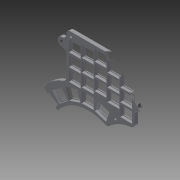
# Autodesk Inventor part: 20kb rebuild Printable Left
Saved by Autodesk Inventor 2015 SP2 (Build 190223200, 223)
## iProperties
Created: 2016-01-05
Part Number: 20kb rebuild Printable Left
Material: Generic
Document SubType Name: Modeling
Designer: Josh
Density: 1 g/cm^3
Appearance: Default
Author: Josh
Autodesk Inventor part; units mm, degrees
(part 1 of 2)
ref_plane "YZ Plane" through (0, 0, 0) normal (1, 0, 0) x (0, 1, 0)
ref_plane "XZ Plane" through (0, 0, 0) normal (0, 1, 0) x (-1, 0, 0)
ref_plane "XY Plane" through (0, 0, 0) normal (0, 0, 1) x (1, 0, 0)
sketch "Sketch1" plane through (0, 0, 0) normal (0, 0, 1) x (1, 0, 0)
  line L0 (4.268, -29.8985) -> (3.518, -29.8985) projected
  line L1 (3.518, -29.8985) -> (3.518, -30.4985) projected
  line L2 (3.518, -30.4985) -> (-10.482, -30.4985) projected
  line L3 (-10.482, -30.4985) -> (-10.482, -29.8985) projected
  line L4 (-10.482, -29.8985) -> (-11.232, -29.8985) projected
  line L5 (-11.232, -29.8985) -> (-11.232, -17.0985) projected
  line L6 (-11.232, -17.0985) -> (-10.482, -17.0985) projected
  line L7 (-10.482, -17.0985) -> (-10.482, -16.4985) projected
  line L8 (-10.482, -16.4985) -> (3.518, -16.4985) projected
  line L9 (3.518, -16.4985) -> (3.518, -17.0985) projected
  line L10 (3.518, -17.0985) -> (4.268, -17.0985) projected
  line L11 (4.268, -17.0985) -> (4.268, -29.8985) projected
  line L12 (26.884, -23.4145) -> (27.5924, -23.661) projected
  line L13 (27.5924, -23.661) -> (23.3854, -35.7499) projected
  line L14 (23.3854, -35.7499) -> (22.6771, -35.5034) projected
  line L15 (22.6771, -35.5034) -> (22.4799, -36.0701) projected
  line L16 (22.4799, -36.0701) -> (9.2576, -31.4687) projected
  line L17 (9.2576, -31.4687) -> (9.4548, -30.902) projected
  line L18 (9.4548, -30.902) -> (8.7465, -30.6555) projected
  line L19 (8.7465, -30.6555) -> (12.9535, -18.5666) projected
  line L20 (12.9535, -18.5666) -> (13.6618, -18.8131) projected
  line L21 (13.6618, -18.8131) -> (13.859, -18.2465) projected
  line L22 (13.859, -18.2465) -> (27.0812, -22.8479) projected
  line L23 (27.0812, -22.8479) -> (26.884, -23.4145) projected
  line L24 (-15.7105, -30.6555) -> (-16.4188, -30.902) projected
  line L25 (-16.4188, -30.902) -> (-16.2216, -31.4687) projected
  line L26 (-16.2216, -31.4687) -> (-29.4438, -36.0701) projected
  line L27 (-29.4438, -36.0701) -> (-29.641, -35.5034) projected
  line L28 (-29.641, -35.5034) -> (-30.3494, -35.7499) projected
  line L29 (-30.3494, -35.7499) -> (-34.5564, -23.661) projected
  line L30 (-34.5564, -23.661) -> (-33.848, -23.4145) projected
  line L31 (-33.848, -23.4145) -> (-34.0452, -22.8479) projected
  line L32 (-34.0452, -22.8479) -> (-20.823, -18.2465) projected
  line L33 (-20.823, -18.2465) -> (-20.6258, -18.8131) projected
  line L34 (-20.6258, -18.8131) -> (-19.9175, -18.5666) projected
  line L35 (-19.9175, -18.5666) -> (-15.7105, -30.6555) projected
  line L36 (-34.3302, -37.9368) -> (-34.9182, -38.4024) projected
  line L37 (-34.9182, -38.4024) -> (-34.5457, -38.8728) projected
  line L38 (-34.5457, -38.8728) -> (-45.521, -47.5643) projected
  line L39 (-45.521, -47.5643) -> (-45.8935, -47.0939) projected
  line L40 (-45.8935, -47.0939) -> (-46.4815, -47.5596) projected
  line L41 (-46.4815, -47.5596) -> (-54.428, -37.525) projected
  line L42 (-54.428, -37.525) -> (-53.84, -37.0594) projected
  line L43 (-53.84, -37.0594) -> (-54.2125, -36.589) projected
  line L44 (-54.2125, -36.589) -> (-43.2372, -27.8975) projected
  line L45 (-43.2372, -27.8975) -> (-42.8647, -28.3679) projected
  line L46 (-42.8647, -28.3679) -> (-42.2768, -27.9022) projected
  line L47 (-42.2768, -27.9022) -> (-34.3302, -37.9368) projected
  line L48 (-49.5224, -50.9334) -> (-49.9247, -51.5664) projected
  line L49 (-49.9247, -51.5664) -> (-49.4183, -51.8882) projected
  line L50 (-49.4183, -51.8882) -> (-56.9272, -63.7041) projected
  line L51 (-56.9272, -63.7041) -> (-57.4336, -63.3823) projected
  line L52 (-57.4336, -63.3823) -> (-57.8359, -64.0153) projected
  line L53 (-57.8359, -64.0153) -> (-68.639, -57.15) projected
  line L54 (-68.639, -57.15) -> (-68.2367, -56.517) projected
  line L55 (-68.2367, -56.517) -> (-68.7431, -56.1952) projected
  line L56 (-68.7431, -56.1952) -> (-61.2342, -44.3793) projected
  line L57 (-61.2342, -44.3793) -> (-60.7278, -44.7011) projected
  line L58 (-60.7278, -44.7011) -> (-60.3256, -44.0681) projected
  line L59 (-60.3256, -44.0681) -> (-49.5224, -50.9334) projected
  line L60 (-15.532, 38.9932) -> (-14.782, 38.9932) projected
  line L61 (-14.782, 38.9932) -> (-14.782, 26.1932) projected
  line L62 (-14.782, 26.1932) -> (-15.532, 26.1932) projected
  line L63 (-15.532, 26.1932) -> (-15.532, 25.5932) projected
  line L64 (-15.532, 25.5932) -> (-29.532, 25.5932) projected
  line L65 (-29.532, 25.5932) -> (-29.532, 26.1932) projected
  line L66 (-29.532, 26.1932) -> (-30.282, 26.1932) projected
  line L67 (-30.282, 26.1932) -> (-30.282, 38.9932) projected
  line L68 (-30.282, 38.9932) -> (-29.532, 38.9932) projected
  line L69 (-29.532, 38.9932) -> (-29.532, 39.5932) projected
  line L70 (-29.532, 39.5932) -> (-15.532, 39.5932) projected
  line L71 (-15.532, 39.5932) -> (-15.532, 38.9932) projected
  line L72 (3.518, 41.3744) -> (4.268, 41.3744) projected
  line L73 (4.268, 41.3744) -> (4.268, 28.5744) projected
  line L74 (4.268, 28.5744) -> (3.518, 28.5744) projected
  line L75 (3.518, 28.5744) -> (3.518, 27.9744) projected
  line L76 (3.518, 27.9744) -> (-10.482, 27.9744) projected
  line L77 (-10.482, 27.9744) -> (-10.482, 28.5744) projected
  line L78 (-10.482, 28.5744) -> (-11.232, 28.5744) projected
  line L79 (-11.232, 28.5744) -> (-11.232, 41.3744) projected
  line L80 (-11.232, 41.3744) -> (-10.482, 41.3744) projected
  line L81 (-10.482, 41.3744) -> (-10.482, 41.9744) projected
  line L82 (-10.482, 41.9744) -> (3.518, 41.9744) projected
  line L83 (3.518, 41.9744) -> (3.518, 41.3744) projected
  line L84 (60.668, 31.8494) -> (61.418, 31.8494) projected
  line L85 (61.418, 31.8494) -> (61.418, 19.0494) projected
  line L86 (61.418, 19.0494) -> (60.668, 19.0494) projected
  line L87 (60.668, 19.0494) -> (60.668, 18.4494) projected
  line L88 (60.668, 18.4494) -> (46.668, 18.4494) projected
  line L89 (46.668, 18.4494) -> (46.668, 19.0494) projected
  line L90 (46.668, 19.0494) -> (45.918, 19.0494) projected
  line L91 (45.918, 19.0494) -> (45.918, 31.8494) projected
  line L92 (45.918, 31.8494) -> (46.668, 31.8494) projected
  line L93 (46.668, 31.8494) -> (46.668, 32.4494) projected
  line L94 (46.668, 32.4494) -> (60.668, 32.4494) projected
  line L95 (60.668, 32.4494) -> (60.668, 31.8494) projected
  line L96 (22.568, 46.1369) -> (23.318, 46.1369) projected
  line L97 (23.318, 46.1369) -> (23.318, 33.3369) projected
  line L98 (23.318, 33.3369) -> (22.568, 33.3369) projected
  line L99 (22.568, 33.3369) -> (22.568, 32.7369) projected
  line L100 (22.568, 32.7369) -> (8.568, 32.7369) projected
  line L101 (8.568, 32.7369) -> (8.568, 33.3369) projected
  line L102 (8.568, 33.3369) -> (7.818, 33.3369) projected
  line L103 (7.818, 33.3369) -> (7.818, 46.1369) projected
  line L104 (7.818, 46.1369) -> (8.568, 46.1369) projected
  line L105 (8.568, 46.1369) -> (8.568, 46.7369) projected
  line L106 (8.568, 46.7369) -> (22.568, 46.7369) projected
  line L107 (22.568, 46.7369) -> (22.568, 46.1369) projected
  line L108 (41.618, 41.3744) -> (42.368, 41.3744) projected
  line L109 (42.368, 41.3744) -> (42.368, 28.5744) projected
  line L110 (42.368, 28.5744) -> (41.618, 28.5744) projected
  line L111 (41.618, 28.5744) -> (41.618, 27.9744) projected
  line L112 (41.618, 27.9744) -> (27.618, 27.9744) projected
  line L113 (27.618, 27.9744) -> (27.618, 28.5744) projected
  line L114 (27.618, 28.5744) -> (26.868, 28.5744) projected
  line L115 (26.868, 28.5744) -> (26.868, 41.3744) projected
  line L116 (26.868, 41.3744) -> (27.618, 41.3744) projected
  line L117 (27.618, 41.3744) -> (27.618, 41.9744) projected
  line L118 (27.618, 41.9744) -> (41.618, 41.9744) projected
  line L119 (41.618, 41.9744) -> (41.618, 41.3744) projected
  line L120 (-15.532, 19.9432) -> (-14.782, 19.9432) projected
  line L121 (-14.782, 19.9432) -> (-14.782, 7.1432) projected
  line L122 (-14.782, 7.1432) -> (-15.532, 7.1432) projected
  line L123 (-15.532, 7.1432) -> (-15.532, 6.5432) projected
  line L124 (-15.532, 6.5432) -> (-29.532, 6.5432) projected
  line L125 (-29.532, 6.5432) -> (-29.532, 7.1432) projected
  line L126 (-29.532, 7.1432) -> (-30.282, 7.1432) projected
  line L127 (-30.282, 7.1432) -> (-30.282, 19.9432) projected
  line L128 (-30.282, 19.9432) -> (-29.532, 19.9432) projected
  line L129 (-29.532, 19.9432) -> (-29.532, 20.5432) projected
  line L130 (-29.532, 20.5432) -> (-15.532, 20.5432) projected
  line L131 (-15.532, 20.5432) -> (-15.532, 19.9432) projected
  line L132 (3.518, 22.3244) -> (4.268, 22.3244) projected
  line L133 (4.268, 22.3244) -> (4.268, 9.5244) projected
  line L134 (4.268, 9.5244) -> (3.518, 9.5244) projected
  line L135 (3.518, 9.5244) -> (3.518, 8.9244) projected
  line L136 (3.518, 8.9244) -> (-10.482, 8.9244) projected
  line L137 (-10.482, 8.9244) -> (-10.482, 9.5244) projected
  line L138 (-10.482, 9.5244) -> (-11.232, 9.5244) projected
  line L139 (-11.232, 9.5244) -> (-11.232, 22.3244) projected
  line L140 (-11.232, 22.3244) -> (-10.482, 22.3244) projected
  line L141 (-10.482, 22.3244) -> (-10.482, 22.9244) projected
  line L142 (-10.482, 22.9244) -> (3.518, 22.9244) projected
  line L143 (3.518, 22.9244) -> (3.518, 22.3244) projected
  line L144 (60.668, 12.7994) -> (61.418, 12.7994) projected
  line L145 (61.418, 12.7994) -> (61.418, -0.0006) projected
  line L146 (61.418, -0.0006) -> (60.668, -0.0006) projected
  line L147 (60.668, -0.0006) -> (60.668, -0.6006) projected
  line L148 (60.668, -0.6006) -> (46.668, -0.6006) projected
  line L149 (46.668, -0.6006) -> (46.668, -0.0006) projected
  line L150 (46.668, -0.0006) -> (45.918, -0.0006) projected
  line L151 (45.918, -0.0006) -> (45.918, 12.7994) projected
  line L152 (45.918, 12.7994) -> (46.668, 12.7994) projected
  line L153 (46.668, 12.7994) -> (46.668, 13.3994) projected
  line L154 (46.668, 13.3994) -> (60.668, 13.3994) projected
  line L155 (60.668, 13.3994) -> (60.668, 12.7994) projected
  line L156 (22.568, 27.0869) -> (23.318, 27.0869) projected
  line L157 (23.318, 27.0869) -> (23.318, 14.2869) projected
  line L158 (23.318, 14.2869) -> (22.568, 14.2869) projected
  line L159 (22.568, 14.2869) -> (22.568, 13.6869) projected
  line L160 (22.568, 13.6869) -> (8.568, 13.6869) projected
  line L161 (8.568, 13.6869) -> (8.568, 14.2869) projected
  line L162 (8.568, 14.2869) -> (7.818, 14.2869) projected
  line L163 (7.818, 14.2869) -> (7.818, 27.0869) projected
  line L164 (7.818, 27.0869) -> (8.568, 27.0869) projected
  line L165 (8.568, 27.0869) -> (8.568, 27.6869) projected
  line L166 (8.568, 27.6869) -> (22.568, 27.6869) projected
  line L167 (22.568, 27.6869) -> (22.568, 27.0869) projected
  line L168 (41.618, 22.3244) -> (42.368, 22.3244) projected
  line L169 (42.368, 22.3244) -> (42.368, 9.5244) projected
  line L170 (42.368, 9.5244) -> (41.618, 9.5244) projected
  line L171 (41.618, 9.5244) -> (41.618, 8.9244) projected
  line L172 (41.618, 8.9244) -> (27.618, 8.9244) projected
  line L173 (27.618, 8.9244) -> (27.618, 9.5244) projected
  line L174 (27.618, 9.5244) -> (26.868, 9.5244) projected
  line L175 (26.868, 9.5244) -> (26.868, 22.3244) projected
  line L176 (26.868, 22.3244) -> (27.618, 22.3244) projected
  line L177 (27.618, 22.3244) -> (27.618, 22.9244) projected
  line L178 (27.618, 22.9244) -> (41.618, 22.9244) projected
  line L179 (41.618, 22.9244) -> (41.618, 22.3244) projected
  line L180 (42.368, -9.5256) -> (41.618, -9.5256) projected
  line L181 (41.618, -9.5256) -> (41.618, -10.1256) projected
  line L182 (41.618, -10.1256) -> (27.618, -10.1256) projected
  line L183 (27.618, -10.1256) -> (27.618, -9.5256) projected
  line L184 (27.618, -9.5256) -> (26.868, -9.5256) projected
  line L185 (26.868, -9.5256) -> (26.868, 3.2744) projected
  line L186 (26.868, 3.2744) -> (27.618, 3.2744) projected
  line L187 (27.618, 3.2744) -> (27.618, 3.8744) projected
  line L188 (27.618, 3.8744) -> (41.618, 3.8744) projected
  line L189 (41.618, 3.8744) -> (41.618, 3.2744) projected
  line L190 (41.618, 3.2744) -> (42.368, 3.2744) projected
  line L191 (42.368, 3.2744) -> (42.368, -9.5256) projected
  line L192 (23.318, -4.7631) -> (22.568, -4.7631) projected
  line L193 (22.568, -4.7631) -> (22.568, -5.3631) projected
  line L194 (22.568, -5.3631) -> (8.568, -5.3631) projected
  line L195 (8.568, -5.3631) -> (8.568, -4.7631) projected
  line L196 (8.568, -4.7631) -> (7.818, -4.7631) projected
  line L197 (7.818, -4.7631) -> (7.818, 8.0369) projected
  line L198 (7.818, 8.0369) -> (8.568, 8.0369) projected
  line L199 (8.568, 8.0369) -> (8.568, 8.6369) projected
  line L200 (8.568, 8.6369) -> (22.568, 8.6369) projected
  line L201 (22.568, 8.6369) -> (22.568, 8.0369) projected
  line L202 (22.568, 8.0369) -> (23.318, 8.0369) projected
  line L203 (23.318, 8.0369) -> (23.318, -4.7631) projected
  line L204 (61.418, -19.0506) -> (60.668, -19.0506) projected
  line L205 (60.668, -19.0506) -> (60.668, -19.6506) projected
  line L206 (60.668, -19.6506) -> (46.668, -19.6506) projected
  line L207 (46.668, -19.6506) -> (46.668, -19.0506) projected
  line L208 (46.668, -19.0506) -> (45.918, -19.0506) projected
  line L209 (45.918, -19.0506) -> (45.918, -6.2506) projected
  line L210 (45.918, -6.2506) -> (46.668, -6.2506) projected
  line L211 (46.668, -6.2506) -> (46.668, -5.6506) projected
  line L212 (46.668, -5.6506) -> (60.668, -5.6506) projected
  line L213 (60.668, -5.6506) -> (60.668, -6.2506) projected
  line L214 (60.668, -6.2506) -> (61.418, -6.2506) projected
  line L215 (61.418, -6.2506) -> (61.418, -19.0506) projected
  line L216 (4.268, -9.5256) -> (3.518, -9.5256) projected
  line L217 (3.518, -9.5256) -> (3.518, -10.1256) projected
  line L218 (3.518, -10.1256) -> (-10.482, -10.1256) projected
  line L219 (-10.482, -10.1256) -> (-10.482, -9.5256) projected
  line L220 (-10.482, -9.5256) -> (-11.232, -9.5256) projected
  line L221 (-11.232, -9.5256) -> (-11.232, 3.2744) projected
  line L222 (-11.232, 3.2744) -> (-10.482, 3.2744) projected
  line L223 (-10.482, 3.2744) -> (-10.482, 3.8744) projected
  line L224 (-10.482, 3.8744) -> (3.518, 3.8744) projected
  line L225 (3.518, 3.8744) -> (3.518, 3.2744) projected
  line L226 (3.518, 3.2744) -> (4.268, 3.2744) projected
  line L227 (4.268, 3.2744) -> (4.268, -9.5256) projected
  line L228 (-14.782, -11.9068) -> (-15.532, -11.9068) projected
  line L229 (-15.532, -11.9068) -> (-15.532, -12.5068) projected
  line L230 (-15.532, -12.5068) -> (-29.532, -12.5068) projected
  line L231 (-29.532, -12.5068) -> (-29.532, -11.9068) projected
  line L232 (-29.532, -11.9068) -> (-30.282, -11.9068) projected
  line L233 (-30.282, -11.9068) -> (-30.282, 0.8932) projected
  line L234 (-30.282, 0.8932) -> (-29.532, 0.8932) projected
  line L235 (-29.532, 0.8932) -> (-29.532, 1.4932) projected
  line L236 (-29.532, 1.4932) -> (-15.532, 1.4932) projected
  line L237 (-15.532, 1.4932) -> (-15.532, 0.8932) projected
  line L238 (-15.532, 0.8932) -> (-14.782, 0.8932) projected
  line L239 (-14.782, 0.8932) -> (-14.782, -11.9068) projected
  arc A0 (66.368, 46.0869) -> (60.018, 52.4369) centre (60.018, 46.0869) ccw projected
  line L240 (-28.882, 52.4369) -> (60.018, 52.4369) projected
  arc A1 (-28.882, 52.4369) -> (-35.232, 46.0869) centre (-28.882, 46.0869) ccw projected
  line L241 (-35.232, -10.3249) -> (-35.232, 46.0869) projected
  arc A2 (-39.5057, -16.3259) -> (-35.232, -10.3249) centre (-41.582, -10.3249) ccw projected
  arc A3 (-39.5057, -16.3259) -> (-76.6111, -57.9488) centre (-20.8194, -70.3346) ccw projected
  arc A4 (22.0394, -41.2849) -> (29.0899, -40.1547) centre (24.7335, -35.5347) ccw projected
  arc A5 (60.6824, -25.6489) -> (29.0899, -40.1547) centre (66.368, -79.6875) ccw projected
  arc A6 (60.6824, -25.6489) -> (66.368, -19.3337) centre (60.018, -19.3337) ccw projected
  line L242 (66.368, 46.0869) -> (66.368, -19.3337) projected
  line L243 (-15.5241, 49.2404) -> (-15.124, 49.2404) construction
  line L244 (-15.124, 49.2404) -> (-16.3541, 46.1109) construction
  line L245 (-16.3541, 46.1109) -> (-16.7666, 46.1109) construction
  line L246 (-16.7666, 46.1109) -> (-16.3565, 47.0643) construction
  line L247 (-16.3565, 47.0643) -> (-17.1865, 49.2404) construction
  line L248 (-17.1865, 49.2404) -> (-16.7715, 49.2404) construction
  line L249 (-16.7715, 49.2404) -> (-16.1466, 47.546) construction
  line L250 (-16.1466, 47.546) -> (-15.5241, 49.2404) construction
  spline S0 degree 2 poles (-20.9606, 46.9729) (-21.0693, 46.9433) (-21.2916, 46.9087) (-21.388, 46.9087) knots 0 0 0 1 2 2 2 construction
  spline S1 degree 2 poles (-21.388, 46.9087) (-21.7016, 46.9087) (-22.0549, 47.2669) (-22.0549, 47.6546) knots 0 0 0 1 2 2 2 construction
  line L251 (-22.0549, 47.6546) -> (-22.0549, 48.9218) construction
  line L252 (-22.0549, 48.9218) -> (-22.3142, 48.9218) construction
  line L253 (-22.3142, 48.9218) -> (-22.3142, 49.2404) construction
  line L254 (-22.3142, 49.2404) -> (-22.0549, 49.2404) construction
  line L255 (-22.0549, 49.2404) -> (-22.0549, 49.8974) construction
  line L256 (-22.0549, 49.8974) -> (-21.6695, 49.8974) construction
  line L257 (-21.6695, 49.8974) -> (-21.6695, 49.2404) construction
  line L258 (-21.6695, 49.2404) -> (-20.9606, 49.2404) construction
  line L259 (-20.9606, 49.2404) -> (-20.9606, 48.9218) construction
  line L260 (-20.9606, 48.9218) -> (-21.6695, 48.9218) construction
  line L261 (-21.6695, 48.9218) -> (-21.6695, 47.8325) construction
  spline S2 degree 2 poles (-21.6695, 47.8325) (-21.6695, 47.6596) (-21.6572, 47.4694) (-21.6152, 47.3879) knots 0 0 0 1 2 2 2 construction
  spline S3 degree 2 poles (-21.6152, 47.3879) (-21.5806, 47.3163) (-21.425, 47.2446) (-21.2916, 47.2446) knots 0 0 0 1 2 2 2 construction
  spline S4 degree 2 poles (-21.2916, 47.2446) (-21.1978, 47.2446) (-21.0224, 47.3014) (-20.9829, 47.3187) knots 0 0 0 1 2 2 2 construction
  line L262 (-20.9829, 47.3187) -> (-20.9606, 47.3187) construction
  line L263 (-20.9606, 47.3187) -> (-20.9606, 46.9729) construction
  line L264 (-27.4568, 46.9532) -> (-27.8619, 46.9532) construction
  line L265 (-27.8619, 46.9532) -> (-27.8619, 49.6405) construction
  line L266 (-27.8619, 49.6405) -> (-28.8845, 49.6405) construction
  line L267 (-28.8845, 49.6405) -> (-28.8845, 50.0012) construction
  line L268 (-28.8845, 50.0012) -> (-26.4342, 50.0012) construction
  line L269 (-26.4342, 50.0012) -> (-26.4342, 49.6405) construction
  line L270 (-26.4342, 49.6405) -> (-27.4568, 49.6405) construction
  line L271 (-27.4568, 49.6405) -> (-27.4568, 46.9532) construction
  spline S5 degree 2 poles (53.9938, 46.8371) (53.8851, 46.8074) (53.6628, 46.7728) (53.5664, 46.7728) knots 0 0 0 1 2 2 2 construction
  spline S6 degree 2 poles (53.5664, 46.7728) (53.2527, 46.7728) (52.8995, 47.131) (52.8995, 47.5188) knots 0 0 0 1 2 2 2 construction
  line L272 (52.8995, 47.5188) -> (52.8995, 48.7859) construction
  line L273 (52.8995, 48.7859) -> (52.6402, 48.7859) construction
  line L274 (52.6402, 48.7859) -> (52.6402, 49.1045) construction
  line L275 (52.6402, 49.1045) -> (52.8995, 49.1045) construction
  line L276 (52.8995, 49.1045) -> (52.8995, 49.7616) construction
  line L277 (52.8995, 49.7616) -> (53.2849, 49.7616) construction
  line L278 (53.2849, 49.7616) -> (53.2849, 49.1045) construction
  line L279 (53.2849, 49.1045) -> (53.9938, 49.1045) construction
  line L280 (53.9938, 49.1045) -> (53.9938, 48.7859) construction
  line L281 (53.9938, 48.7859) -> (53.2849, 48.7859) construction
  line L282 (53.2849, 48.7859) -> (53.2849, 47.6966) construction
  spline S7 degree 2 poles (53.2849, 47.6966) (53.2849, 47.5237) (53.2972, 47.3335) (53.3392, 47.252) knots 0 0 0 1 2 2 2 construction
  spline S8 degree 2 poles (53.3392, 47.252) (53.3738, 47.1804) (53.5294, 47.1088) (53.6628, 47.1088) knots 0 0 0 1 2 2 2 construction
  spline S9 degree 2 poles (53.6628, 47.1088) (53.7566, 47.1088) (53.932, 47.1656) (53.9715, 47.1829) knots 0 0 0 1 2 2 2 construction
  line L283 (53.9715, 47.1829) -> (53.9938, 47.1829) construction
  line L284 (53.9938, 47.1829) -> (53.9938, 46.8371) construction
  line L285 (52.3092, 49.1045) -> (52.3092, 46.8173) construction
  line L286 (52.3092, 46.8173) -> (51.9239, 46.8173) construction
  line L287 (51.9239, 46.8173) -> (51.9239, 49.1045) construction
  line L288 (51.9239, 49.1045) -> (52.3092, 49.1045) construction
  spline S10 degree 2 poles (48.7376, 47.0347) (48.5918, 46.8914) (48.2065, 46.7531) (47.9249, 46.7531) knots 0 0 0 1 2 2 2 construction
  spline S11 degree 2 poles (47.9249, 46.7531) (47.6557, 46.7531) (47.2555, 46.8939) (47.1148, 47.0347) knots 0 0 0 1 2 2 2 construction
  spline S12 degree 2 poles (47.1148, 47.0347) (46.9542, 47.1927) (46.8233, 47.6374) (46.8233, 47.9634) knots 0 0 0 1 2 2 2 construction
  line L289 (46.8233, 47.9634) -> (46.8233, 49.8653) construction
  line L290 (46.8233, 49.8653) -> (47.2284, 49.8653) construction
  line L291 (47.2284, 49.8653) -> (47.2284, 47.9634) construction
  spline S13 degree 2 poles (47.2284, 47.9634) (47.2284, 47.751) (47.2827, 47.4645) (47.3593, 47.3484) knots 0 0 0 1 2 2 2 construction
  spline S14 degree 2 poles (47.3593, 47.3484) (47.4408, 47.2249) (47.7224, 47.0989) (47.9249, 47.0989) knots 0 0 0 1 2 2 2 construction
  spline S15 degree 2 poles (47.9249, 47.0989) (48.1151, 47.0989) (48.4115, 47.2249) (48.493, 47.3484) knots 0 0 0 1 2 2 2 construction
  spline S16 degree 2 poles (48.493, 47.3484) (48.5696, 47.4645) (48.6239, 47.7485) (48.6239, 47.9535) knots 0 0 0 1 2 2 2 construction
  line L292 (48.6239, 47.9535) -> (48.6239, 49.8653) construction
  line L293 (48.6239, 49.8653) -> (49.029, 49.8653) construction
  line L294 (49.029, 49.8653) -> (49.029, 47.9634) construction
  spline S17 degree 2 poles (49.029, 47.9634) (49.029, 47.6448) (48.9006, 47.1903) (48.7376, 47.0347) knots 0 0 0 1 2 2 2 construction
  line L295 (44.9634, 50.0012) -> (44.9634, 46.8173) construction
  line L296 (44.9634, 46.8173) -> (44.5781, 46.8173) construction
  line L297 (44.5781, 46.8173) -> (44.5781, 47.0495) construction
  spline S18 degree 2 poles (44.5781, 47.0495) (44.4891, 46.9754) (44.3582, 46.8766) (44.2693, 46.8346) knots 0 0 0 1 2 2 2 construction
  spline S19 degree 2 poles (44.2693, 46.8346) (44.1878, 46.7951) (44.0124, 46.7531) (43.8963, 46.7531) knots 0 0 0 1 2 2 2 construction
  spline S20 degree 2 poles (43.8963, 46.7531) (43.7086, 46.7531) (43.3924, 46.9087) (43.2813, 47.0594) knots 0 0 0 1 2 2 2 construction
  spline S21 degree 2 poles (43.2813, 47.0594) (43.1701, 47.21) (43.0466, 47.6546) (43.0466, 47.9436) knots 0 0 0 1 2 2 2 construction
  spline S22 degree 2 poles (43.0466, 47.9436) (43.0466, 48.245) (43.2023, 48.6846) (43.3381, 48.8501) knots 0 0 0 1 2 2 2 construction
  spline S23 degree 2 poles (43.3381, 48.8501) (43.4641, 48.9983) (43.8173, 49.1688) (44.0124, 49.1688) knots 0 0 0 1 2 2 2 construction
  spline S24 degree 2 poles (44.0124, 49.1688) (44.1828, 49.1688) (44.4373, 49.0922) (44.5781, 49.0132) knots 0 0 0 1 2 2 2 construction
  line L298 (44.5781, 49.0132) -> (44.5781, 50.0012) construction
  line L299 (44.5781, 50.0012) -> (44.9634, 50.0012) construction
  line L300 (34.2089, 49.1045) -> (34.6091, 49.1045) construction
  line L301 (34.6091, 49.1045) -> (33.379, 45.975) construction
  line L302 (33.379, 45.975) -> (32.9665, 45.975) construction
  line L303 (32.9665, 45.975) -> (33.3765, 46.9285) construction
  line L304 (33.3765, 46.9285) -> (32.5466, 49.1045) construction
  line L305 (32.5466, 49.1045) -> (32.9616, 49.1045) construction
  line L306 (32.9616, 49.1045) -> (33.5865, 47.4101) construction
  line L307 (33.5865, 47.4101) -> (34.2089, 49.1045) construction
  spline S25 degree 2 poles (32.0328, 46.8297) (31.9217, 46.7975) (31.7389, 46.7654) (31.6006, 46.7654) knots 0 0 0 1 2 2 2 construction
  spline S26 degree 2 poles (31.6006, 46.7654) (31.0522, 46.7654) (30.4496, 47.3805) (30.4496, 47.9486) knots 0 0 0 1 2 2 2 construction
  spline S27 degree 2 poles (30.4496, 47.9486) (30.4496, 48.5068) (31.035, 49.1688) (31.5067, 49.1688) knots 0 0 0 1 2 2 2 construction
  spline S28 degree 2 poles (31.5067, 49.1688) (31.7191, 49.1688) (32.0477, 49.0453) (32.1687, 48.9144) knots 0 0 0 1 2 2 2 construction
  spline S29 degree 2 poles (32.1687, 48.9144) (32.2922, 48.7834) (32.4231, 48.4055) (32.4231, 48.1314) knots 0 0 0 1 2 2 2 construction
  line L308 (32.4231, 48.1314) -> (32.4231, 47.9214) construction
  line L309 (32.4231, 47.9214) -> (30.8398, 47.9214) construction
  spline S30 degree 2 poles (30.8398, 47.9214) (30.8398, 47.5237) (31.24, 47.1014) (31.5956, 47.1014) knots 0 0 0 1 2 2 2 construction
  spline S31 degree 2 poles (31.5956, 47.1014) (31.7216, 47.1014) (31.9661, 47.1582) (32.0649, 47.2026) knots 0 0 0 1 2 2 2 construction
  spline S32 degree 2 poles (32.0649, 47.2026) (32.1687, 47.252) (32.312, 47.3385) (32.3589, 47.378) knots 0 0 0 1 2 2 2 construction
  line L310 (32.3589, 47.378) -> (32.3811, 47.378) construction
  line L311 (32.3811, 47.378) -> (32.3811, 46.9581) construction
  spline S33 degree 2 poles (32.3811, 46.9581) (32.3144, 46.9309) (32.1119, 46.8519) (32.0328, 46.8297) knots 0 0 0 1 2 2 2 construction
  line L312 (29.0589, 48.5043) -> (30.3952, 46.8173) construction
  line L313 (30.3952, 46.8173) -> (29.8691, 46.8173) construction
  line L314 (29.8691, 46.8173) -> (28.7551, 48.2351) construction
  line L315 (28.7551, 48.2351) -> (28.5773, 48.035) construction
  line L316 (28.5773, 48.035) -> (28.5773, 46.8173) construction
  line L317 (28.5773, 46.8173) -> (28.1722, 46.8173) construction
  line L318 (28.1722, 46.8173) -> (28.1722, 49.8653) construction
  line L319 (28.1722, 49.8653) -> (28.5773, 49.8653) construction
  line L320 (28.5773, 49.8653) -> (28.5773, 48.4648) construction
  line L321 (28.5773, 48.4648) -> (29.8271, 49.8653) construction
  line L322 (29.8271, 49.8653) -> (30.3211, 49.8653) construction
  line L323 (30.3211, 49.8653) -> (29.0589, 48.5043) construction
  spline S34 degree 2 poles (35.9849, 49.1688) (36.3727, 49.1688) (36.8173, 48.5488) (36.8173, 47.998) knots 0 0 0 1 2 2 2 construction
  spline S35 degree 2 poles (36.8173, 47.998) (36.8173, 47.4373) (36.2739, 46.7531) (35.8638, 46.7531) knots 0 0 0 1 2 2 2 construction
  spline S36 degree 2 poles (35.8638, 46.7531) (35.6786, 46.7531) (35.4143, 46.8445) (35.2859, 46.9235) knots 0 0 0 1 2 2 2 construction
  line L324 (35.2859, 46.9235) -> (35.2612, 46.8173) construction
  line L325 (35.2612, 46.8173) -> (34.9005, 46.8173) construction
  line L326 (34.9005, 46.8173) -> (34.9005, 50.0012) construction
  line L327 (34.9005, 50.0012) -> (35.2859, 50.0012) construction
  line L328 (35.2859, 50.0012) -> (35.2859, 48.865) construction
  spline S37 degree 2 poles (35.2859, 48.865) (35.4316, 48.9959) (35.77, 49.1688) (35.9849, 49.1688) knots 0 0 0 1 2 2 2 construction
  spline S38 degree 2 poles (38.077, 49.1688) (38.5413, 49.1688) (39.0971, 48.5364) (39.0971, 47.9609) knots 0 0 0 1 2 2 2 construction
  spline S39 degree 2 poles (39.0971, 47.9609) (39.0971, 47.3829) (38.5413, 46.7531) (38.077, 46.7531) knots 0 0 0 1 2 2 2 construction
  spline S40 degree 2 poles (38.077, 46.7531) (37.6003, 46.7531) (37.0544, 47.4027) (37.0544, 47.9609) knots 0 0 0 1 2 2 2 construction
  spline S41 degree 2 poles (37.0544, 47.9609) (37.0544, 48.534) (37.6175, 49.1688) (38.077, 49.1688) knots 0 0 0 1 2 2 2 construction
  line L329 (40.7668, 46.8173) -> (40.7668, 47.0594) construction
  spline S42 degree 2 poles (40.7668, 47.0594) (40.7199, 47.0248) (40.5618, 46.9013) (40.4877, 46.8642) knots 0 0 0 1 2 2 2 construction
  spline S43 degree 2 poles (40.4877, 46.8642) (40.3864, 46.8099) (40.1962, 46.7531) (40.0233, 46.7531) knots 0 0 0 1 2 2 2 construction
  spline S44 degree 2 poles (40.0233, 46.7531) (39.8826, 46.7531) (39.6281, 46.8593) (39.5318, 46.9556) knots 0 0 0 1 2 2 2 construction
  spline S45 degree 2 poles (39.5318, 46.9556) (39.4404, 47.0495) (39.3293, 47.3261) (39.3293, 47.4793) knots 0 0 0 1 2 2 2 construction
  spline S46 degree 2 poles (39.3293, 47.4793) (39.3293, 47.7164) (39.5293, 48.0523) (39.7467, 48.1486) knots 0 0 0 1 2 2 2 construction
  spline S47 degree 2 poles (39.7467, 48.1486) (39.9394, 48.2376) (40.463, 48.3043) (40.7668, 48.3215) knots 0 0 0 1 2 2 2 construction
  line L330 (40.7668, 48.3215) -> (40.7668, 48.3956) construction
  spline S48 degree 2 poles (40.7668, 48.3956) (40.7668, 48.529) (40.6853, 48.6945) (40.6112, 48.7414) knots 0 0 0 1 2 2 2 construction
  spline S49 degree 2 poles (40.6112, 48.7414) (40.5371, 48.7884) (40.3247, 48.818) (40.2111, 48.818) knots 0 0 0 1 2 2 2 construction
  spline S50 degree 2 poles (40.2111, 48.818) (40.0777, 48.818) (39.7171, 48.739) (39.5367, 48.6624) knots 0 0 0 1 2 2 2 construction
  line L331 (39.5367, 48.6624) -> (39.5145, 48.6624) construction
  line L332 (39.5145, 48.6624) -> (39.5145, 49.0551) construction
  spline S51 degree 2 poles (39.5145, 49.0551) (39.6207, 49.0848) (40.0184, 49.1589) (40.2135, 49.1589) knots 0 0 0 1 2 2 2 construction
  spline S52 degree 2 poles (40.2135, 49.1589) (40.4507, 49.1589) (40.7742, 49.0848) (40.9027, 48.9885) knots 0 0 0 1 2 2 2 construction
  spline S53 degree 2 poles (40.9027, 48.9885) (41.0286, 48.8946) (41.1521, 48.5957) (41.1521, 48.3808) knots 0 0 0 1 2 2 2 construction
  line L333 (41.1521, 48.3808) -> (41.1521, 46.8173) construction
  line L334 (41.1521, 46.8173) -> (40.7668, 46.8173) construction
  line L335 (42.9059, 49.0922) -> (42.9059, 48.692) construction
  line L336 (42.9059, 48.692) -> (42.8861, 48.692) construction
  spline S54 degree 2 poles (42.8861, 48.692) (42.8416, 48.7044) (42.7453, 48.7093) (42.6786, 48.7093) knots 0 0 0 1 2 2 2 construction
  spline S55 degree 2 poles (42.6786, 48.7093) (42.523, 48.7093) (42.2167, 48.5735) (42.0784, 48.4401) knots 0 0 0 1 2 2 2 construction
  line L337 (42.0784, 48.4401) -> (42.0784, 46.8173) construction
  line L338 (42.0784, 46.8173) -> (41.6931, 46.8173) construction
  line L339 (41.6931, 46.8173) -> (41.6931, 49.1045) construction
  line L340 (41.6931, 49.1045) -> (42.0784, 49.1045) construction
  line L341 (42.0784, 49.1045) -> (42.0784, 48.7637) construction
  spline S56 degree 2 poles (42.0784, 48.7637) (42.2883, 48.9514) (42.602, 49.1045) (42.7502, 49.1045) knots 0 0 0 1 2 2 2 construction
  spline S57 degree 2 poles (42.7502, 49.1045) (42.8095, 49.1045) (42.8688, 49.0996) (42.9059, 49.0922) knots 0 0 0 1 2 2 2 construction
  line L342 (51.3755, 48.3018) -> (51.3755, 46.8173) construction
  line L343 (51.3755, 46.8173) -> (50.9902, 46.8173) construction
  line L344 (50.9902, 46.8173) -> (50.9902, 48.1215) construction
  spline S58 degree 2 poles (50.9902, 48.1215) (50.9902, 48.2796) (50.9606, 48.5513) (50.9161, 48.6328) knots 0 0 0 1 2 2 2 construction
  spline S59 degree 2 poles (50.9161, 48.6328) (50.8692, 48.7192) (50.7012, 48.8032) (50.558, 48.8032) knots 0 0 0 1 2 2 2 construction
  spline S60 degree 2 poles (50.558, 48.8032) (50.4147, 48.8032) (50.1109, 48.6501) (49.9652, 48.5266) knots 0 0 0 1 2 2 2 construction
  line L345 (49.9652, 48.5266) -> (49.9652, 46.8173) construction
  line L346 (49.9652, 46.8173) -> (49.5798, 46.8173) construction
  line L347 (49.5798, 46.8173) -> (49.5798, 49.1045) construction
  line L348 (49.5798, 49.1045) -> (49.9652, 49.1045) construction
  line L349 (49.9652, 49.1045) -> (49.9652, 48.8501) construction
  spline S61 degree 2 poles (49.9652, 48.8501) (50.1381, 49.0057) (50.4715, 49.1688) (50.6592, 49.1688) knots 0 0 0 1 2 2 2 construction
  spline S62 degree 2 poles (50.6592, 49.1688) (50.9952, 49.1688) (51.3755, 48.7242) (51.3755, 48.3018) knots 0 0 0 1 2 2 2 construction
  line L350 (52.3364, 49.8851) -> (52.3364, 49.4849) construction
  line L351 (52.3364, 49.4849) -> (51.8992, 49.4849) construction
  line L352 (51.8992, 49.4849) -> (51.8992, 49.8851) construction
  line L353 (51.8992, 49.8851) -> (52.3364, 49.8851) construction
  spline S63 degree 2 poles (56.4539, 49.9271) (56.9553, 49.9271) (57.4271, 49.1367) (57.4271, 48.3413) knots 0 0 0 1 2 2 2 construction
  spline S64 degree 2 poles (57.4271, 48.3413) (57.4271, 47.5213) (56.9504, 46.7531) (56.4539, 46.7531) knots 0 0 0 1 2 2 2 construction
  spline S65 degree 2 poles (56.4539, 46.7531) (55.95, 46.7531) (55.4782, 47.5361) (55.4782, 48.3388) knots 0 0 0 1 2 2 2 construction
  spline S66 degree 2 poles (55.4782, 48.3388) (55.4782, 49.1638) (55.9549, 49.9271) (56.4539, 49.9271) knots 0 0 0 1 2 2 2 construction
  line L354 (59.697, 47.1705) -> (59.697, 46.8173) construction
  line L355 (59.697, 46.8173) -> (57.8173, 46.8173) construction
  line L356 (57.8173, 46.8173) -> (57.8173, 47.2496) construction
  spline S67 degree 2 poles (57.8173, 47.2496) (58.0199, 47.4398) (58.3805, 47.793) (58.5534, 47.9832) knots 0 0 0 1 2 2 2 construction
  spline S68 degree 2 poles (58.5534, 47.9832) (58.9017, 48.366) (59.1561, 48.8254) (59.1561, 49.07) knots 0 0 0 1 2 2 2 construction
  spline S69 degree 2 poles (59.1561, 49.07) (59.1561, 49.1984) (59.077, 49.3911) (59.0054, 49.4528) knots 0 0 0 1 2 2 2 construction
  spline S70 degree 2 poles (59.0054, 49.4528) (58.9338, 49.5146) (58.7461, 49.5763) (58.6324, 49.5763) knots 0 0 0 1 2 2 2 construction
  spline S71 degree 2 poles (58.6324, 49.5763) (58.5238, 49.5763) (58.3015, 49.522) (58.2002, 49.48) knots 0 0 0 1 2 2 2 construction
  spline S72 degree 2 poles (58.2002, 49.48) (58.1137, 49.4454) (57.9532, 49.3466) (57.9038, 49.312) knots 0 0 0 1 2 2 2 construction
  line L357 (57.9038, 49.312) -> (57.8816, 49.312) construction
  line L358 (57.8816, 49.312) -> (57.8816, 49.7467) construction
  spline S73 degree 2 poles (57.8816, 49.7467) (58.0075, 49.8085) (58.4595, 49.9295) (58.6621, 49.9295) knots 0 0 0 1 2 2 2 construction
  spline S74 degree 2 poles (58.6621, 49.9295) (59.0894, 49.9295) (59.5711, 49.4775) (59.5711, 49.0922) knots 0 0 0 1 2 2 2 construction
  spline S75 degree 2 poles (59.5711, 49.0922) (59.5711, 48.9119) (59.4871, 48.6105) (59.413, 48.4821) knots 0 0 0 1 2 2 2 construction
  spline S76 degree 2 poles (59.413, 48.4821) (59.3389, 48.3487) (59.124, 48.0869) (59.0054, 47.9609) knots 0 0 0 1 2 2 2 construction
  spline S77 degree 2 poles (59.0054, 47.9609) (58.8128, 47.751) (58.341, 47.3014) (58.2002, 47.1705) knots 0 0 0 1 2 2 2 construction
  line L359 (58.2002, 47.1705) -> (59.697, 47.1705) construction
  spline S78 degree 2 poles (-24.7299, 46.9655) (-24.841, 46.9334) (-25.0238, 46.9013) (-25.1621, 46.9013) knots 0 0 0 1 2 2 2 construction
  spline S79 degree 2 poles (-25.1621, 46.9013) (-25.7105, 46.9013) (-26.3132, 47.5163) (-26.3132, 48.0844) knots 0 0 0 1 2 2 2 construction
  spline S80 degree 2 poles (-26.3132, 48.0844) (-26.3132, 48.6426) (-25.7278, 49.3046) (-25.256, 49.3046) knots 0 0 0 1 2 2 2 construction
  spline S81 degree 2 poles (-25.256, 49.3046) (-25.0436, 49.3046) (-24.7151, 49.1811) (-24.594, 49.0502) knots 0 0 0 1 2 2 2 construction
  spline S82 degree 2 poles (-24.594, 49.0502) (-24.4705, 48.9193) (-24.3396, 48.5414) (-24.3396, 48.2672) knots 0 0 0 1 2 2 2 construction
  line L360 (-24.3396, 48.2672) -> (-24.3396, 48.0573) construction
  line L361 (-24.3396, 48.0573) -> (-25.9229, 48.0573) construction
  spline S83 degree 2 poles (-25.9229, 48.0573) (-25.9229, 47.6596) (-25.5228, 47.2372) (-25.1671, 47.2372) knots 0 0 0 1 2 2 2 construction
  spline S84 degree 2 poles (-25.1671, 47.2372) (-25.0411, 47.2372) (-24.7966, 47.294) (-24.6978, 47.3385) knots 0 0 0 1 2 2 2 construction
  spline S85 degree 2 poles (-24.6978, 47.3385) (-24.594, 47.3879) (-24.4508, 47.4743) (-24.4038, 47.5139) knots 0 0 0 1 2 2 2 construction
  line L362 (-24.4038, 47.5139) -> (-24.3816, 47.5139) construction
  line L363 (-24.3816, 47.5139) -> (-24.3816, 47.0939) construction
  spline S86 degree 2 poles (-24.3816, 47.0939) (-24.4483, 47.0668) (-24.6508, 46.9877) (-24.7299, 46.9655) knots 0 0 0 1 2 2 2 construction
  spline S87 degree 2 poles (-22.6674, 47.1063) (-22.7885, 47.005) (-23.0972, 46.8988) (-23.3319, 46.8988) knots 0 0 0 1 2 2 2 construction
  spline S88 degree 2 poles (-23.3319, 46.8988) (-23.5616, 46.8988) (-23.9592, 47.0223) (-24.0902, 47.0915) knots 0 0 0 1 2 2 2 construction
  line L364 (-24.0902, 47.0915) -> (-24.0902, 47.5237) construction
  line L365 (-24.0902, 47.5237) -> (-24.0704, 47.5237) construction
  spline S89 degree 2 poles (-24.0704, 47.5237) (-24.021, 47.4842) (-23.8876, 47.3904) (-23.7765, 47.3385) knots 0 0 0 1 2 2 2 construction
  spline S90 degree 2 poles (-23.7765, 47.3385) (-23.6801, 47.2916) (-23.443, 47.2224) (-23.317, 47.2224) knots 0 0 0 1 2 2 2 construction
  spline S91 degree 2 poles (-23.317, 47.2224) (-23.2256, 47.2224) (-23.0157, 47.2644) (-22.9663, 47.299) knots 0 0 0 1 2 2 2 construction
  spline S92 degree 2 poles (-22.9663, 47.299) (-22.8947, 47.3459) (-22.8304, 47.4521) (-22.8304, 47.5608) knots 0 0 0 1 2 2 2 construction
  spline S93 degree 2 poles (-22.8304, 47.5608) (-22.8304, 47.6966) (-22.9786, 47.8374) (-23.1688, 47.8844) knots 0 0 0 1 2 2 2 construction
  spline S94 degree 2 poles (-23.1688, 47.8844) (-23.2429, 47.9016) (-23.4801, 47.951) (-23.5813, 47.9782) knots 0 0 0 1 2 2 2 construction
  spline S95 degree 2 poles (-23.5813, 47.9782) (-23.8432, 48.0548) (-24.0803, 48.3709) (-24.0803, 48.5957) knots 0 0 0 1 2 2 2 construction
  spline S96 degree 2 poles (-24.0803, 48.5957) (-24.0803, 48.9069) (-23.6134, 49.2947) (-23.2281, 49.2947) knots 0 0 0 1 2 2 2 construction
  spline S97 degree 2 poles (-23.2281, 49.2947) (-23.0379, 49.2947) (-22.6526, 49.2009) (-22.5217, 49.1292) knots 0 0 0 1 2 2 2 construction
  line L366 (-22.5217, 49.1292) -> (-22.5217, 48.7167) construction
  line L367 (-22.5217, 48.7167) -> (-22.5415, 48.7167) construction
  spline S98 degree 2 poles (-22.5415, 48.7167) (-22.6897, 48.8353) (-23.0503, 48.9712) (-23.2355, 48.9712) knots 0 0 0 1 2 2 2 construction
  spline S99 degree 2 poles (-23.2355, 48.9712) (-23.4257, 48.9712) (-23.6875, 48.8106) (-23.6875, 48.6501) knots 0 0 0 1 2 2 2 construction
  spline S100 degree 2 poles (-23.6875, 48.6501) (-23.6875, 48.5043) (-23.5319, 48.3635) (-23.359, 48.3191) knots 0 0 0 1 2 2 2 construction
  spline S101 degree 2 poles (-23.359, 48.3191) (-23.275, 48.2968) (-23.0626, 48.2524) (-22.9465, 48.2252) knots 0 0 0 1 2 2 2 construction
  spline S102 degree 2 poles (-22.9465, 48.2252) (-22.6946, 48.161) (-22.4377, 47.8671) (-22.4377, 47.6127) knots 0 0 0 1 2 2 2 construction
  spline S103 degree 2 poles (-22.4377, 47.6127) (-22.4377, 47.4645) (-22.5538, 47.2026) (-22.6674, 47.1063) knots 0 0 0 1 2 2 2 construction
  line L368 (-18.2214, 46.9532) -> (-18.6265, 46.9532) construction
  line L369 (-18.6265, 46.9532) -> (-18.6265, 49.6405) construction
  line L370 (-18.6265, 49.6405) -> (-19.6491, 49.6405) construction
  line L371 (-19.6491, 49.6405) -> (-19.6491, 50.0012) construction
  line L372 (-19.6491, 50.0012) -> (-17.1988, 50.0012) construction
  line L373 (-17.1988, 50.0012) -> (-17.1988, 49.6405) construction
  line L374 (-17.1988, 49.6405) -> (-18.2214, 49.6405) construction
  line L375 (-18.2214, 49.6405) -> (-18.2214, 46.9532) construction
  spline S104 degree 2 poles (-13.7482, 49.3046) (-13.3555, 49.3046) (-12.9158, 48.6822) (-12.9158, 48.1585) knots 0 0 0 1 2 2 2 construction
  spline S105 degree 2 poles (-12.9158, 48.1585) (-12.9158, 47.5855) (-13.4617, 46.9087) (-13.8791, 46.9087) knots 0 0 0 1 2 2 2 construction
  spline S106 degree 2 poles (-13.8791, 46.9087) (-14.0495, 46.9087) (-14.3114, 46.9877) (-14.4472, 47.0692) knots 0 0 0 1 2 2 2 construction
  line L376 (-14.4472, 47.0692) -> (-14.4472, 46.1109) construction
  line L377 (-14.4472, 46.1109) -> (-14.8325, 46.1109) construction
  line L378 (-14.8325, 46.1109) -> (-14.8325, 49.2404) construction
  line L379 (-14.8325, 49.2404) -> (-14.4472, 49.2404) construction
  line L380 (-14.4472, 49.2404) -> (-14.4472, 49.0008) construction
  spline S107 degree 2 poles (-14.4472, 49.0008) (-14.304, 49.1317) (-13.9532, 49.3046) (-13.7482, 49.3046) knots 0 0 0 1 2 2 2 construction
  spline S108 degree 2 poles (-11.0905, 46.9655) (-11.2016, 46.9334) (-11.3844, 46.9013) (-11.5227, 46.9013) knots 0 0 0 1 2 2 2 construction
  spline S109 degree 2 poles (-11.5227, 46.9013) (-12.0711, 46.9013) (-12.6737, 47.5163) (-12.6737, 48.0844) knots 0 0 0 1 2 2 2 construction
  spline S110 degree 2 poles (-12.6737, 48.0844) (-12.6737, 48.6426) (-12.0883, 49.3046) (-11.6166, 49.3046) knots 0 0 0 1 2 2 2 construction
  spline S111 degree 2 poles (-11.6166, 49.3046) (-11.4042, 49.3046) (-11.0756, 49.1811) (-10.9546, 49.0502) knots 0 0 0 1 2 2 2 construction
  spline S112 degree 2 poles (-10.9546, 49.0502) (-10.8311, 48.9193) (-10.7002, 48.5414) (-10.7002, 48.2672) knots 0 0 0 1 2 2 2 construction
  line L381 (-10.7002, 48.2672) -> (-10.7002, 48.0573) construction
  line L382 (-10.7002, 48.0573) -> (-12.2835, 48.0573) construction
  spline S113 degree 2 poles (-12.2835, 48.0573) (-12.2835, 47.6596) (-11.8833, 47.2372) (-11.5277, 47.2372) knots 0 0 0 1 2 2 2 construction
  spline S114 degree 2 poles (-11.5277, 47.2372) (-11.4017, 47.2372) (-11.1571, 47.294) (-11.0583, 47.3385) knots 0 0 0 1 2 2 2 construction
  spline S115 degree 2 poles (-11.0583, 47.3385) (-10.9546, 47.3879) (-10.8113, 47.4743) (-10.7644, 47.5139) knots 0 0 0 1 2 2 2 construction
  line L383 (-10.7644, 47.5139) -> (-10.7422, 47.5139) construction
  line L384 (-10.7422, 47.5139) -> (-10.7422, 47.0939) construction
  spline S116 degree 2 poles (-10.7422, 47.0939) (-10.8089, 47.0668) (-11.0114, 46.9877) (-11.0905, 46.9655) knots 0 0 0 1 2 2 2 construction
  arc A7 (-76.6111, -57.9488) -> (-57.446, -72.9896) centre (-63.4241, -60.8763) ccw projected
  arc A8 (-57.446, -72.9896) -> (-54.4513, -69.8694) centre (-60.2562, -67.2953) ccw projected
  arc A9 (22.0394, -41.2849) -> (-54.4513, -69.8694) centre (-2.2075, -93.0363) ccw projected
  point P0 (0, 0)
extrude "Extrusion1" add sketch "Sketch1" along normal blind 1.1
sketch "Sketch2" plane through (0, 0, 1.1) normal (0, 0, 1) x (1, 0, 0)
  line L0 (-13.782, 40.5932) -> (-31.282, 40.5932) projected
  line L1 (-31.282, 2.4932) -> (-31.282, -13.5068) projected
  line L2 (-31.282, -13.5068) -> (-13.782, -13.5068) projected
  line L3 (-13.782, -13.5068) -> (-13.782, 2.4932) projected
  line L4 (-13.782, 2.4932) -> (-31.282, 2.4932) projected
  line L5 (24.318, -6.3631) -> (24.318, 9.6369) projected
  line L6 (24.318, 9.6369) -> (6.818, 9.6369) projected
  line L7 (6.818, 9.6369) -> (6.818, -6.3631) projected
  line L8 (6.818, -6.3631) -> (24.318, -6.3631) projected
  line L9 (44.918, -4.6506) -> (44.918, -20.6506) projected
  line L10 (44.918, -20.6506) -> (62.418, -20.6506) projected
  line L11 (62.418, -20.6506) -> (62.418, -4.6506) projected
  line L12 (62.418, -4.6506) -> (44.918, -4.6506) projected
  line L13 (43.368, -11.1256) -> (43.368, 4.8744) projected
  line L14 (43.368, 4.8744) -> (25.868, 4.8744) projected
  line L15 (25.868, 4.8744) -> (25.868, -11.1256) projected
  line L16 (25.868, -11.1256) -> (43.368, -11.1256) projected
  line L17 (5.268, -11.1256) -> (5.268, 4.8744) projected
  line L18 (5.268, 4.8744) -> (-12.232, 4.8744) projected
  line L19 (-12.232, 4.8744) -> (-12.232, -11.1256) projected
  line L20 (-12.232, -11.1256) -> (5.268, -11.1256) projected
  line L21 (43.368, 7.9244) -> (43.368, 23.9244) projected
  line L22 (43.368, 23.9244) -> (25.868, 23.9244) projected
  line L23 (25.868, 23.9244) -> (25.868, 7.9244) projected
  line L24 (25.868, 7.9244) -> (43.368, 7.9244) projected
  line L25 (24.318, 12.6869) -> (24.318, 28.6869) projected
  line L26 (24.318, 28.6869) -> (6.818, 28.6869) projected
  line L27 (6.818, 28.6869) -> (6.818, 12.6869) projected
  line L28 (6.818, 12.6869) -> (24.318, 12.6869) projected
  line L29 (44.918, 14.3994) -> (44.918, -1.6006) projected
  line L30 (44.918, -1.6006) -> (62.418, -1.6006) projected
  line L31 (62.418, -1.6006) -> (62.418, 14.3994) projected
  line L32 (62.418, 14.3994) -> (44.918, 14.3994) projected
  line L33 (5.268, 7.9244) -> (5.268, 23.9244) projected
  line L34 (5.268, 23.9244) -> (-12.232, 23.9244) projected
  line L35 (-12.232, 23.9244) -> (-12.232, 7.9244) projected
  line L36 (-12.232, 7.9244) -> (5.268, 7.9244) projected
  line L37 (-31.282, 21.5432) -> (-31.282, 5.5432) projected
  line L38 (-31.282, 5.5432) -> (-13.782, 5.5432) projected
  line L39 (-13.782, 5.5432) -> (-13.782, 21.5432) projected
  line L40 (-13.782, 21.5432) -> (-31.282, 21.5432) projected
  line L41 (43.368, 26.9744) -> (43.368, 42.9744) projected
  line L42 (43.368, 42.9744) -> (25.868, 42.9744) projected
  line L43 (25.868, 42.9744) -> (25.868, 26.9744) projected
  line L44 (25.868, 26.9744) -> (43.368, 26.9744) projected
  line L45 (24.318, 31.7369) -> (24.318, 47.7369) projected
  line L46 (24.318, 47.7369) -> (6.818, 47.7369) projected
  line L47 (6.818, 47.7369) -> (6.818, 31.7369) projected
  line L48 (6.818, 31.7369) -> (24.318, 31.7369) projected
  line L49 (44.918, 33.4494) -> (44.918, 17.4494) projected
  line L50 (44.918, 17.4494) -> (62.418, 17.4494) projected
  line L51 (62.418, 17.4494) -> (62.418, 33.4494) projected
  line L52 (62.418, 33.4494) -> (44.918, 33.4494) projected
  line L53 (5.268, 26.9744) -> (5.268, 42.9744) projected
  line L54 (5.268, 42.9744) -> (-12.232, 42.9744) projected
  line L55 (-12.232, 42.9744) -> (-12.232, 26.9744) projected
  line L56 (-12.232, 26.9744) -> (5.268, 26.9744) projected
  line L57 (-31.282, 40.5932) -> (-31.282, 24.5932) projected
  line L58 (-31.282, 24.5932) -> (-13.782, 24.5932) projected
  line L59 (-13.782, 24.5932) -> (-13.782, 40.5932) projected
  line L60 (-13.782, 40.5932) -> (-31.282, 40.5932) projected
  line L61 (-36.0267, -22.4786) -> (-30.7679, -37.5897) projected
  line L62 (-30.7679, -37.5897) -> (-14.2402, -31.8379) projected
  line L63 (-14.2402, -31.8379) -> (-19.4989, -16.7268) projected
  line L64 (-19.4989, -16.7268) -> (-36.0267, -22.4786) projected
  line L65 (-70.5257, -57.1358) -> (-57.0218, -65.7174) projected
  line L66 (-57.0218, -65.7174) -> (-47.6357, -50.9475) projected
  line L67 (-47.6357, -50.9475) -> (-61.1396, -42.3659) projected
  line L68 (-61.1396, -42.3659) -> (-70.5257, -57.1358) projected
  line L69 (12.5349, -16.7268) -> (7.2762, -31.8379) projected
  line L70 (7.2762, -31.8379) -> (23.804, -37.5897) projected
  line L71 (23.804, -37.5897) -> (29.0627, -22.4786) projected
  line L72 (29.0627, -22.4786) -> (12.5349, -16.7268) projected
  line L73 (-12.232, -15.4985) -> (-12.232, -31.4985) projected
  line L74 (-12.232, -31.4985) -> (5.268, -31.4985) projected
  line L75 (5.268, -31.4985) -> (5.268, -15.4985) projected
  line L76 (5.268, -15.4985) -> (-12.232, -15.4985) projected
  line L77 (-56.2053, -36.8915) -> (-46.2721, -49.4347) projected
  line L78 (-46.2721, -49.4347) -> (-32.553, -38.5703) projected
  line L79 (-32.553, -38.5703) -> (-42.4861, -26.0271) projected
  line L80 (-42.4861, -26.0271) -> (-56.2053, -36.8915) projected
  arc A0 (66.368, 46.0869) -> (60.018, 52.4369) centre (60.018, 46.0869) ccw projected
  line L81 (66.368, 46.0869) -> (66.368, -19.3337) projected
  arc A1 (60.6824, -25.6489) -> (66.368, -19.3337) centre (60.018, -19.3337) ccw projected
  arc A2 (60.6824, -25.6489) -> (29.0899, -40.1547) centre (66.368, -79.6875) ccw projected
  arc A3 (22.0394, -41.2849) -> (29.0899, -40.1547) centre (24.7335, -35.5347) ccw projected
  arc A4 (-39.5057, -16.3259) -> (-76.6111, -57.9488) centre (-20.8194, -70.3346) ccw projected
  arc A5 (-39.5057, -16.3259) -> (-35.232, -10.3249) centre (-41.582, -10.3249) ccw projected
  line L82 (-35.232, -10.3249) -> (-35.232, 46.0869) projected
  arc A6 (-28.882, 52.4369) -> (-35.232, 46.0869) centre (-28.882, 46.0869) ccw projected
  line L83 (-28.882, 52.4369) -> (60.018, 52.4369) projected
  arc A7 (-76.6111, -57.9488) -> (-57.446, -72.9896) centre (-63.4241, -60.8763) ccw projected
  arc A8 (-57.446, -72.9896) -> (-54.4513, -69.8694) centre (-60.2562, -67.2953) ccw projected
  arc A9 (22.0394, -41.2849) -> (-54.4513, -69.8694) centre (-2.2075, -93.0363) ccw projected
  point P0 (0, 0)
extrude "Extrusion2" add sketch "Sketch2" along normal blind 3.98